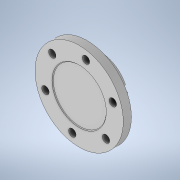
# Autodesk Inventor part: 轴承通盖1
Saved by Autodesk Inventor 2020 (Build 240168000, 168)
## iProperties
Created: 2021-06-16
Part Number: 轴承通盖1
Material: 常规
Document SubType Name: Modeling
Designer: dell
Density: 1 g/cm^3
Appearance: 默认
Author: dell
Autodesk Inventor part; units mm, degrees
ref_plane "YZ Plane" through (0, 0, 0) normal (1, 0, 0) x (0, 1, 0)
ref_plane "XZ Plane" through (0, 0, 0) normal (0, 1, 0) x (-1, 0, 0)
ref_plane "XY Plane" through (0, 0, 0) normal (0, 0, 1) x (1, 0, 0)
ref_plane "工作平面1" through (0, 0, 0) normal (0, 0, 1) x (1, 0, 0)
sketch "草图1" plane through (0, 0, 0) normal (0, 0, 1) x (1, 0, 0)
  arc A0 (32.5, 65) -> (32.5, -65) centre (32.5, 0) ccw construction
  line L0 (32.5, -65) -> (32.5, -40) construction
  arc A1 (32.5, 40) -> (32.5, -40) centre (32.5, 0) ccw construction
  line L1 (32.5, 40) -> (32.5, 65) construction
  circle A2 centre (32.5, 0) radius 65 projected
  circle A3 centre (72.1024, -34.466) radius 5.5 projected
  circle A4 centre (-17.1496, -17.0637) radius 5.5 projected
  circle A5 centre (82.1496, 17.0637) radius 5.5 projected
  circle A6 centre (42.5472, 51.5296) radius 5.5 projected
  circle A7 centre (22.4528, -51.5296) radius 5.5 projected
  circle A8 centre (-7.1024, 34.466) radius 5.5 projected
  circle A9 centre (32.5, 0) radius 65 projected
  circle A10 centre (32.5, 0) radius 40 construction
  point P0 (0, 0)
extrude "拉伸1" add sketch "草图1" along normal blind 12
sketch "草图2" plane through (32.5, 0, 0) normal (0, 0, -1) x (-1, 0, 0)
  circle A0 centre (0, 0) radius 65 construction
  circle A1 centre (0, 0) radius 40
  circle A2 centre (0, 0) radius 35
  point P0 (32.5, 0)
  dimension "d2" = 80
  dimension "d3" = 70
  constraints: 2 centre point, 2 coincident
  measures "d2" diameter of A1
  measures "d3" diameter of A2
extrude "拉伸2" add sketch "草图2" along normal blind 20
sketch "草图3" plane through (32.5, 0, 12) normal (0, 0, 1) x (1, 0, 0)
  circle A0 centre (0, 0) radius 65 construction
  circle A1 centre (0, 0) radius 40
  point P0 (-32.5, 0)
  dimension "d6" = 80
  constraints: 1 centre point, 1 coincident
  measures "d6" diameter of A1
extrude "拉伸3" cut sketch "草图3" against normal blind 1
fillet "圆角1" radius 1 1 edges at (-7.5, 0, 11)
sketch "草图4" plane through (32.5, 0, -20) normal (0, 0, -1) x (-1, 0, 0)
  circle A0 centre (0, 0) radius 35 construction
  circle A1 centre (49.6496, -17.0637) radius 5.5 construction
  circle A2 centre (-49.6496, 17.0637) radius 5.5 construction
  line L0 (49.6496, -17.0637) -> (-49.6496, 17.0637) construction
  line L1 (66.9706, -27.2462) -> (-94.2998, 28.1795)
  line L2 (-94.2998, 28.1795) -> (-91.6996, 35.7451)
  line L3 (-91.6996, 35.7451) -> (69.5708, -19.6806)
  line L4 (69.5708, -19.6806) -> (66.9706, -27.2462)
  point P0 (32.5, 0)
  dimension "d10" = 8
  constraints: 10 end point, 3 perpendicular, 1 other
  measures "d10" distance of L1.end L2.end
extrude "拉伸4" cut sketch "草图4" against normal blind 8
ref_plane "工作平面2" through (-0.3829, -11.3012, -12) normal (-0.3250221, 0.9457064, 0) x (0.9457064, 0.3250221, 0)
